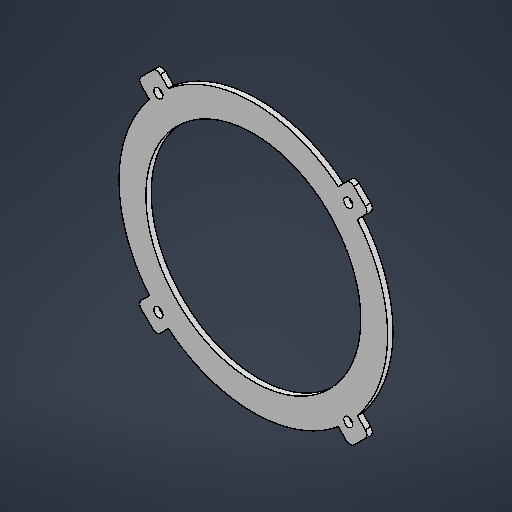
# Autodesk Inventor part: Succ_Plate
Saved by Autodesk Inventor 2026.1 (Build 301233000, 233)
## iProperties
Created: 2025-11-18
Part Number: Succ_Plate
Material: Generic
Document SubType Name: Modeling
Designer: 1char
Mass: 6.05518 g
Surface Area: 73.5774 cm^2
Volume: 6.05518 cm^3
Density: 1 g/cm^3
Appearance: Default
Author: 1char
Autodesk Inventor part; units mm, degrees
ref_plane "YZ Plane" through (0, 0, 0) normal (1, 0, 0) x (0, 1, 0)
ref_plane "XZ Plane" through (0, 0, 0) normal (0, 1, 0) x (-1, 0, 0)
ref_plane "XY Plane" through (0, 0, 0) normal (0, 0, 1) x (1, 0, 0)
sketch "Sketch1" plane through (0, 0, 0) normal (0, 1, 0) x (-1, 0, 0)
  circle A0 centre (0, 0) radius 40
  circle A1 centre (0, 0) radius 50
  dimension "d0" = 80
  dimension "d1" = 100
  constraints: 2 centre point, 2 coincident
  measures "d0" diameter of A0
  measures "d1" diameter of A1
extrude "Extrusion1" add sketch "Sketch1" along normal blind 2
sketch "Sketch2" plane through (0, 0, 0) normal (0, 1, 0) x (-1, 0, 0)
  line L0 (0, 0) -> (-39.598, 39.598) construction
  circle A0 centre (0, 0) radius 50 construction
  line L1 (-31.6426, 38.7137) -> (-36.0624, 43.1335)
  line L2 (-36.0624, 43.1335) -> (-39.598, 39.598)
  line L3 (70, 0) -> (-70, 0) construction
  line L4 (-38.7137, 31.6426) -> (-43.1335, 36.0624)
  line L5 (-43.1335, 36.0624) -> (-39.598, 39.598)
  arc A1 (-31.6426, 38.7137) -> (-38.7137, 31.6426) centre (0, 0) ccw
  dimension "d4" = 56
  dimension "d6" = 5
  dimension "d7" = 45
  constraints: 10 end point, 2 perpendicular, 2 point on circle, 2 symmetric about line, 1 centre point, 3 other
  measures "d4" distance of L0.start L0.end
  measures "d6" distance of L1.end L0.end
  measures "d7" angle of L0 L3
extrude "Extrusion2" add sketch "Sketch2" along normal blind 2
fillet "Fillet1" radius 2 2 edges at (43.1335, 1, 36.0624) (36.0624, 1, 43.1335)
sketch "Sketch3" plane through (0, 0, 0) normal (0, -1, 0) x (1, 0, 0)
  line L0 (0, 0) -> (39.598, 39.598) construction
  line L1 (37.4767, 41.7193) -> (41.7193, 37.4767) construction
  point P0 (35.3553, 35.3553)
  dimension "d11" = 50
  constraints: 2 end point, 1 midpoint, 1 point on line
  measures "d11" distance of point (35.355, 35.355) L0.start
hole "Hole1" at (35.3553, 0, 35.3553) direction (0, 1, 0) diameter 3.4 end through all clearance for "Countersunk Flat Head Screw ISO 2009/7046" size "M3" standard "ISO"
pattern_circular "Circular Pattern1" count 4 over 360 about axis through (0, -10, 0) along (0, 1, 0) of "Hole1", "Fillet1", "Extrusion2"
body "Solid1"
